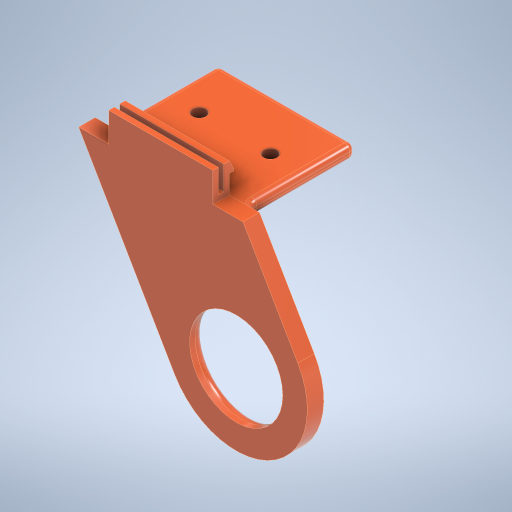
# Autodesk Inventor part: sol arka bacak
Saved by Autodesk Inventor 2023.2 (Build 272271000, 271)
## iProperties
Created: 2022-11-26
Part Number: sol arka bacak
Material: Generic
Document SubType Name: Modeling
Designer: omrfrkmll
Density: 1 g/cm^3
Appearance: Smooth - Light Orange
Author: omrfrkmll
Autodesk Inventor part; units mm, degrees
ref_plane "YZ Plane" through (0, 0, 0) normal (1, 0, 0) x (0, 1, 0)
ref_plane "XZ Plane" through (0, 0, 0) normal (0, 1, 0) x (-1, 0, 0)
ref_plane "XY Plane" through (0, 0, 0) normal (0, 0, 1) x (1, 0, 0)
sketch "Sketch1" plane through (0, 0, 0) normal (0, 0, 1) x (1, 0, 0)
  line L0 (-7.2387, 0) -> (8.5548, 0) construction
  line L1 (0, 6.9097) -> (0, -7.979)
  line L2 (-15, 0) -> (15, 0)
  line L3 (15, 0) -> (57.438, -73.5048)
  line L4 (-15, 0) -> (34.938, -86.4952)
  circle A0 centre (46.188, -80) radius 12.9904
  line L5 (-9.5, 0) -> (9.5, 0)
  line L6 (9.5, 0) -> (9.5, 3.4)
  line L7 (9.5, 3.4) -> (-9.5, 3.4)
  line L8 (-9.5, 3.4) -> (-9.5, 0)
  point P0 (0, 0)
  point P1 (9.5, 0)
  dimension "d0" = 30
  dimension "d1" = 60
  dimension "d2" = 0
  dimension "d3" = 80
  dimension "d4" = 19
  dimension "d5" = 3.4
  constraints: 18 end point, 4 horizontal, 3 parallel, 2 point on circle, 2 tangent, 2 vertical, 1 centre point, 1 perpendicular, 1 point on line, 1 symmetric about line, 2 other
  measures "d0" distance of L2.start L2.end
  measures "d1" angle of L2 L3
  measures "d2" distance between parallel lines of L2 L0
  measures "d3" distance from line of A0.centre L2
  measures "d4" distance between parallel lines of L6 L8
  measures "d5" distance between parallel lines of L2 L7
extrude "Extrusion1" add sketch "Sketch1" along normal mid plane 3
sketch "Sketch2" plane through (0, 0, 1.5) normal (0, 0, 1) x (1, 0, 0)
  arc A0 (34.938, -86.4952) -> (57.438, -73.5048) centre (46.188, -80) ccw projected
  point P0 (0, 0)
  constraints: 1 coincident
hole "Hole1" at (46.188, -80, 1.5) direction (0, 0, -1) diameter 5.6 end through all
sketch "Sketch3" plane through (9.5, 0, 1.5) normal (1, 0, 0) x (0, 0, -1)
  line L0 (0, 0) -> (0, 3.4) projected
  line L1 (0, 3.4) -> (3, 3.4)
  line L2 (3, 3.4) -> (3, 5.4)
  line L3 (3, 5.4) -> (0, 5.4)
  line L4 (0, 5.4) -> (0, 3.4)
  line L5 (3.8, 3.4) -> (3, 3.4)
  line L6 (3.8, 3.4) -> (3.8, 3.8)
  line L7 (3.8, 3.8) -> (3, 5.4)
  point P0 (1.5, 0)
  dimension "d15" = 2
  dimension "d16" = 0.8
  dimension "d44" = 0.4
  constraints: 14 end point, 2 horizontal, 2 parallel, 1 perpendicular, 1 vertical
  measures "d15" distance between parallel lines of L1 L3
  measures "d16" distance from line of L2 L5.start
  measures "d44" distance from line of L5 L6.end
extrude "Extrusion2" add sketch "Sketch3" against normal up to surface (19 mm away)
sketch "Sketch4" plane through (9.5, 0, 1.5) normal (1, 0, 0) x (0, 0, -1)
  line L0 (3, 5.4) -> (0, 5.4) projected
  line L1 (1.5, 5.4) -> (1.5, 1.2343)
  line L2 (1, 5.4916) -> (2, 5.4916)
  line L3 (2, 5.4916) -> (2, 1)
  line L4 (2, 1) -> (1, 1)
  line L5 (1, 1) -> (1, 5.4916)
  line L6 (3, 0) -> (0, 0) projected
  point P0 (1.5, 0)
  point P1 (2, 5.4)
  point P2 (1, 5.4)
  dimension "d19" = 1
  dimension "d20" = 1
  constraints: 10 end point, 2 parallel, 1 horizontal, 1 midpoint, 1 perpendicular, 1 vertical, 1 other
  measures "d19" distance between parallel lines of L6 L4
  measures "d20" distance between parallel lines of L3 L5
extrude "Extrusion3" cut sketch "Sketch4" against normal up to surface (19 mm away) contours L3 L4 L5 L0
sketch "Sketch6" plane through (0, 0, -1.5) normal (0, 0, -1) x (-1, 0, 0)
  line L0 (-15, 0) -> (-57.438, -73.5048) projected
  arc A0 (-24.9985, -17.3179) -> (-2.4985, -30.3083) centre (-13.7485, -23.8131) ccw
  line L1 (15, 0) -> (-34.938, -86.4952) projected
  circle A1 centre (-13.7485, -23.8131) radius 8.5
  line L2 (-57.438, -73.5048) -> (-15, 0) projected
  line L3 (-24.9985, -17.3179) -> (-65.3187, -87.1545)
  line L4 (-65.3187, -87.1545) -> (-42.2173, -99.1033)
  line L5 (-42.2173, -99.1033) -> (-2.4985, -30.3083)
  point P0 (0, 0)
  dimension "d42" = 17
  constraints: 6 end point, 3 tangent, 2 centre point, 2 point on circle, 2 point on line, 1 coincident, 1 collinear
  measures "d42" diameter of A1
extrude "Extrusion5" cut sketch "Sketch6" against normal up to surface (3 mm away)
sketch "Sketch9" plane through (0, 0, -1.5) normal (0, 0, -1) x (-1, 0, 0)
  line L0 (-12.5, -0.2) -> (12.5, -0.2)
  line L1 (12.5, -0.2) -> (12.5, -2.7)
  line L2 (12.5, -2.7) -> (-12.5, -2.7)
  line L3 (-12.5, -2.7) -> (-12.5, -0.2)
  line L4 (-9.5, 3.4) -> (-9.5, 0) projected
  line L5 (9.5, 0) -> (9.5, 3.4) projected
  point P0 (0, 0)
  point P1 (-12.5, -1.45)
  dimension "d37" = 0.2
  dimension "d39" = 2.5
  dimension "d46" = 3
  dimension "d47" = 3
  constraints: 8 end point, 2 parallel, 1 horizontal, 1 midpoint, 1 perpendicular
  measures "d37" distance from line of L0 point (0, 0)
  measures "d39" distance between parallel lines of L2 L0
  measures "d46" distance between parallel lines of L5 L1
  measures "d47" distance between parallel lines of L4 L3
extrude "Extrusion7" add sketch "Sketch9" along normal blind 20
fillet "Fillet2" radius 2 1 edges at (22.2485, -23.8131, -1.5)
fillet "Fillet3" radius 2 3 edges at (-12.5, -1.45, -1.5) (0, -2.7, -1.5) (12.5, -1.45, -1.5)
fillet "Fillet4" radius 1 12 edges at (13.0858, -3.2858, -2.0858) (12.5, -2.7, -12.5) (13.0858, -0.2, -2.0858) (12.5, -0.2, -12.5) (12.5, -1.45, -21.5) (0, -2.7, -21.5) (-12.6552, -2.8552, -2.7276) (-12.5, -2.7, -12.5) (-12.5, -1.45, -21.5) (0, -0.2, -21.5) (-13.0858, -0.2, -2.0858) (-12.5, -0.2, -12.5)
sketch "Sketch10" plane through (-11.5, -2.7, -20.5) normal (0, -1, 0) x (1, 0, 0)
  line L0 (0, 0) -> (23, 0) projected
  line L1 (11.5, 0) -> (11.5, 12.9617)
  line L2 (0, 17) -> (0, 0) projected
  line L3 (0, 8.5) -> (18.4738, 8.5)
  point P0 (11.5, 20.5)
  point P1 (18, 8.5)
  point P2 (5, 8.5)
  dimension "d50" = 13
  constraints: 4 end point, 2 midpoint, 2 point on line, 1 horizontal, 1 symmetric about line, 1 vertical
  measures "d50" distance of point (5, 8.5) point (18, 8.5)
hole "Hole2" at (6.5, -2.7, -12) at (-6.5, -2.7, -12) direction (0, 1, 0) diameter 2.5 depth 2.5
body "Solid1"
